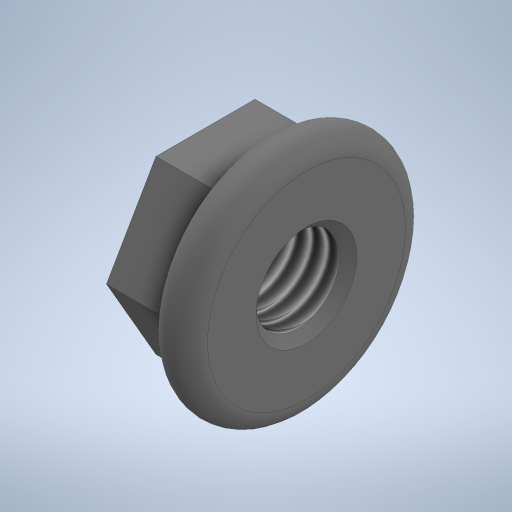
# Autodesk Inventor part: ansi
Saved by Autodesk Inventor 2024 (Build 280153000, 153)
## iProperties
Created: 2023-06-26
Part Number: ansi
Material: Generic
Document SubType Name: Modeling
Designer: _Astitva_Aryan_
Density: 1 g/cm^3
Appearance: Default
Author: _Astitva_Aryan_
Autodesk Inventor part; units mm, degrees
ref_plane "YZ Plane" through (0, 0, 0) normal (1, 0, 0) x (0, 1, 0)
ref_plane "XZ Plane" through (0, 0, 0) normal (0, 1, 0) x (-1, 0, 0)
ref_plane "XY Plane" through (0, 0, 0) normal (0, 0, 1) x (1, 0, 0)
sketch "Sketch1" plane through (0, 0, 0) normal (0, 0, 1) x (1, 0, 0)
  line L0 (0, 7.3391) -> (0, -1.2232) projected
  line L1 (-3.2472, 0) -> (0.765, 0) projected
  line L2 (-2.674, 0) -> (-2.674, 4)
  line L3 (-1, 0) -> (-1, 4.9) construction
  arc A0 (0, 4.9) -> (-1.866, 5.4) centre (-1, 4.9) ccw
  line L4 (-1, 4.9) -> (-1.866, 5.4) construction
  line L5 (-1, 4.9) -> (0, 4.9) construction
  line L6 (-1.866, 5.4) -> (-2.674, 4)
  point P0 (0, 0)
  dimension "d4" = 1
  constraints: 10 end point, 3 coincident, 3 point on line, 2 point on circle, 2 vertical, 1 centre point, 1 equal length, 1 horizontal
  measures "d4" radius of A0
revolve "Revolution1" add sketch "Sketch1" angle 360 about axis through (0, 0, 0) along (1, 0, 0)
ref_plane "Work Plane1" through (0, 0, 0) normal (1, 0, 0) x (0, 0, -1)
sketch "Sketch2" plane through (0, 0, 0) normal (1, 0, 0) x (0, 0, -1)
  circle A0 centre (0, 0) radius 4.9
  line L0 (4.9, 0) -> (2.45, -4.2435)
  line L1 (2.45, -4.2435) -> (-2.45, -4.2435)
  line L2 (-2.45, -4.2435) -> (-4.9, 0)
  line L3 (-4.9, 0) -> (-2.45, 4.2435)
  line L4 (-2.45, 4.2435) -> (2.45, 4.2435)
  line L5 (2.45, 4.2435) -> (4.9, 0)
  dimension "d8" = 9.8
  constraints: 12 end point, 2 coincident, 1 horizontal alignment, 15 other
sketch "Sketch3" plane through (0, 0, 0) normal (1, 0, 0) x (0, 0, -1)
  circle A0 centre (0, 0) radius 2.067
  dimension "d9" = 4.134
  constraints: 1 centre point, 1 coincident
  measures "d9" diameter of A0
extrude "Extrusion1" add sketch "Sketch2" against normal blind 5 contours L0 L1 L2 L3 L4 L5
extrude "Extrusion2" cut sketch "Sketch3" against normal blind 5
chamfer "Chamfer1" distance 0.433 angle 45 2 edges at (0, 0, 2.067) (-5, 0, 2.067)
thread "Thread1" size "M5x0.8" class "6H" standard "ANSI Metric M Profile" length 6
scale "Scale1" factors (10, 10, 10) then translate (9, 0, 0) bodies 1
body "Solid1"
